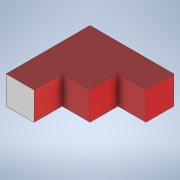
# Autodesk Inventor part: Stair
Saved by Autodesk Inventor 2020 (Build 240168000, 168)
## iProperties
Created: 2019-12-20
Part Number: Stair
Material: Generic
Document SubType Name: Modeling
Designer: Corey
Density: 1 g/cm^3
Appearance: Default
Author: Corey
Autodesk Inventor part; units mm, degrees
ref_plane "YZ Plane" through (0, 0, 0) normal (1, 0, 0) x (0, 1, 0)
ref_plane "XZ Plane" through (0, 0, 0) normal (0, 1, 0) x (-1, 0, 0)
ref_plane "XY Plane" through (0, 0, 0) normal (0, 0, 1) x (1, 0, 0)
sketch "Sketch1" plane through (0, 0, 0) normal (0, 1, 0) x (-1, 0, 0)
  line L0 (0, 0) -> (0, -19.05)
  line L1 (0, -19.05) -> (19.05, -19.05)
  line L2 (19.05, -19.05) -> (19.05, -38.1)
  line L3 (19.05, -38.1) -> (38.1, -38.1)
  line L4 (38.1, -38.1) -> (38.1, -57.15)
  line L5 (38.1, -57.15) -> (57.15, -57.15)
  line L6 (57.15, -57.15) -> (57.15, 0)
  line L7 (57.15, 0) -> (0, 0)
  dimension "d0" = 19.05
  dimension "d1" = 19.05
  dimension "d2" = 19.05
  dimension "d3" = 19.05
  dimension "d4" = 19.05
  dimension "d5" = 19.05
  constraints: 16 end point, 7 perpendicular, 1 vertical
  measures "d0" distance of L0.start L0.end
  measures "d1" distance of L0.end L1.end
  measures "d2" distance of L1.end L2.end
  measures "d3" distance of L2.end L3.end
  measures "d4" distance of L3.end L4.end
  measures "d5" distance of L4.end L5.end
extrude "Extrusion1" add sketch "Sketch1" along normal blind 19.05
body "Solid1"
